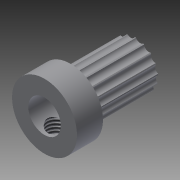
# Autodesk Inventor part: exBolt
Saved by Autodesk Inventor 2013 (Build 170138000, 138)
## iProperties
Created: 2015-01-15
Part Number: exBolt
Material: Generic
Document SubType Name: Modeling
Designer: dzban
Density: 1 g/cm^3
Author: dzban
Autodesk Inventor part; units mm, degrees
ref_plane "YZ Plane" through (0, 0, 0) normal (1, 0, 0) x (0, 1, 0)
ref_plane "XZ Plane" through (0, 0, 0) normal (0, 1, 0) x (-1, 0, 0)
ref_plane "XY Plane" through (0, 0, 0) normal (0, 0, 1) x (1, 0, 0)
sketch "Sketch1" plane through (0, 0, 0) normal (0, 0, 1) x (1, 0, 0)
  line L0 (0, 0.8293) -> (0, 13.3857)
  line L1 (2.5, 0) -> (2.5, 14)
  line L2 (2.5, 14) -> (3.5, 14)
  line L3 (3.5, 14) -> (3.5, 4)
  line L4 (3.5, 4) -> (5, 4)
  line L5 (5, 4) -> (5, 0)
  line L6 (5, 0) -> (2.5, 0)
  point P0 (0, 0)
  dimension "d0" = 2.5
  dimension "d2" = 3.5
  dimension "d3" = 10
  dimension "d4" = 4
  dimension "d5" = 5
  constraints: 14 end point, 3 horizontal, 3 vertical, 1 horizontal alignment, 1 vertical alignment
  measures "d0" distance from line of L1 point (0, 0)
  measures "d2" distance between parallel lines of L3 L0
  measures "d3" distance between parallel lines of L2 L4
  measures "d4" distance between parallel lines of L4 L6
  measures "d5" distance between parallel lines of L0 L5
revolve "Revolution1" add sketch "Sketch1" angle 360 about axis through (0, 0.8293, 0) along (0, 1, 0)
sketch "Sketch2" plane through (0, 0, 0) normal (0, 0, 1) x (1, 0, 0)
  circle A0 centre (0, 2) radius 1.5
  point P0 (0, 0)
  dimension "d7" = 2
  dimension "d8" = 3
  constraints: 1 centre point, 1 vertical alignment
  measures "d7" distance of A0.centre point (0, 0)
  measures "d8" diameter of A0
extrude "Extrusion1" cut sketch "Sketch2" against normal blind 10
thread "Thread1" size "M3x0.5" class "6H" standard "ANSI Metric M Profile" full length
sketch "Sketch3" plane through (0, 14, 0) normal (0, 1, 0) x (1, 0, 0)
  circle A0 centre (0, 0) radius 3.5 projected
  circle A1 centre (0, 3.8726) radius 0.7037
  circle A2 centre (-1.399, 3.6111) radius 0.7037
  circle A3 centre (-2.609, 2.8619) radius 0.7037
  circle A4 centre (-3.4666, 1.7262) radius 0.7037
  circle A5 centre (-3.8561, 0.3573) radius 0.7037
  circle A6 centre (-3.7248, -1.0598) radius 0.7037
  circle A7 centre (-3.0904, -2.3338) radius 0.7037
  circle A8 centre (-2.0387, -3.2926) radius 0.7037
  circle A9 centre (-0.7116, -3.8067) radius 0.7037
  circle A10 centre (0.7116, -3.8067) radius 0.7037
  circle A11 centre (2.0387, -3.2926) radius 0.7037
  circle A12 centre (3.0904, -2.3338) radius 0.7037
  circle A13 centre (3.7248, -1.0598) radius 0.7037
  circle A14 centre (3.8561, 0.3573) radius 0.7037
  circle A15 centre (3.4666, 1.7262) radius 0.7037
  circle A16 centre (2.609, 2.8619) radius 0.7037
  circle A17 centre (1.399, 3.6111) radius 0.7037
  dimension "d15" = 360
  constraints: 17 centre point, 35 other
extrude "Extrusion2" cut sketch "Sketch3" against normal blind 10 contours A0 A14 | A0 A14 | A15 A0 | A0 A15 | A13 A0 | A0 A13 | A16 A0 | A0 A16 | A12 A0 | A0 A12 | A17 A0 | A0 A17 | A11 A0 | A0 A11 | A1 A0 | A0 A1 | A10 A0 | A0 A10 | A2 A0 | A0 A2 | A9 A0 | A0 A9 | A3 A0 | A0 A3 | A8 A0 | A0 A8 | A4 A0 | A0 A4 | A7 A0 | A0 A7 | A5 A0 | A0 A5 | A6 A0 | A0 A6
body "Solid1"
